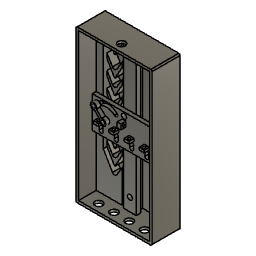
Progetto locker senza bottone v9 (Autodesk Fusion 360 design; units mm, degrees)
Autodesk Fusion 360 part; units mm, degrees
note: some values were not read from the file. Set by a fixed rule: which face or edge a step refers to.
sketch "Schizzo1" plane through (0, 0, 0) normal (0, 1, 0) x (1, 0, 0) in component "Scatola di fissaggio"
  line L0 (-30, -60) -> (30, -60)
  line L1 (30, -60) -> (30, 60)
  line L2 (30, 60) -> (-30, 60)
  line L3 (-30, 60) -> (-30, -60)
  point P0 (0, -60)
  point P1 (-30, 0)
  dimension "d1" = 60
  dimension "d2" = 120
  constraint horizontal L0
  constraint vertical L1
  constraint horizontal L2
  constraint vertical L3
  constraint midpoint L0 P0
  constraint midpoint L3 P1
  constraint vertical origin P0
  constraint horizontal origin P1
  measures "d1" distance of L0.start L0.end
  measures "d2" distance of L0.start L2.end
extrude "Estrusione1" add sketch "Schizzo1" along normal blind 22 makes body 1 in component "Scatola di fissaggio"
shell "Svuotamento1" thickness 2 removed faces 1 at (-10, 0, 20) on bodies 1 in component "Scatola di fissaggio"
ref_plane "Piano di lavoro1" through (0, 10, -58) normal (0, 0, 1) x (1, 0, 0) in component "Guida lineare"
sketch "Schizzo1 (2)" plane through (0, 12.5, -58) normal (0, 0, 1) x (1, 0, 0) in component "Guida lineare"
  line L0 (0, -26.6959) -> (0, 22.9147) construction
  line L1 (0, 0) -> (-5, 0)
  line L2 (-5, 0) -> (-5, 3.5)
  line L3 (-3.5, 5) -> (-2.5, 5)
  line L4 (-2.5, 5) -> (-2.5, 7.5)
  line L5 (28, 7.5) -> (-28, 7.5)
  line L6 (-5, 3.5) -> (-3.5, 5)
  line L7 (0, 0) -> (5, 0)
  line L8 (5, 0) -> (5, 3.5)
  line L9 (5, 3.5) -> (3.5, 5)
  line L10 (3.5, 5) -> (2.5, 5)
  line L11 (2.5, 5) -> (2.5, 7.5)
  point P0 (-5, 5)
  dimension "d7" = 2.5
  dimension "d8" = 5
  dimension "d9" = 5
  dimension "d10" = 2.5
  dimension "d11" = 1.5
  dimension "d12" = 1.5
  constraint vertical L0
  constraint coincident L1.start L0
  constraint coincident L0 L1.start
  constraint perpendicular L0 L1
  constraint perpendicular L1 L2
  constraint perpendicular L2 L3
  constraint perpendicular L3 L4
  constraint coincident L4.end L5
  constraint coincident P0 L2
  constraint coincident P0 L3
  constraint symmetric L0 L1.start L7.start
  constraint symmetric L0 L1.end L7.end
  constraint symmetric L0 L3.end L10.end
  constraint symmetric L0 L4.end L11.end
  constraint symmetric L0 L2.end L8.end
  constraint symmetric L0 L3.start L9.end
  measures "d7" distance of L3.end L4.end
  measures "d8" distance of L1.end P0
  measures "d9" distance of L1.start L1.end
  measures "d10" distance of L0 L4
  measures "d11" distance of P0 L2.end
  measures "d12" distance of P0 L3.start
extrude "Estrusione1'" add sketch "Schizzo1 (2)" along normal up to surface (116 mm away) separate body makes body 2 in component "Guida lineare"
sketch "Schizzo5" plane through (0, 0, 0) normal (0, 0, 1) x (1, 0, 0) in component "Base mobile"
  line L0 (5, 16) -> (3.5, 17.5)
  line L1 (5, 12.5) -> (5, 16)
  line L2 (0, 12.5) -> (5, 12.5)
  line L3 (0, -14.1959) -> (0, 35.4147)
  line L4 (0, 12) -> (5.5, 12)
  line L5 (5.5, 12) -> (5.5, 16.2071)
  line L6 (5.5, 16.2071) -> (3.8536, 17.8536)
  line L7 (3.8536, 17.8536) -> (6.8536, 17.8536)
  line L8 (6.8536, 17.8536) -> (6.8536, 10.8536)
  line L9 (6.8536, 10.8536) -> (0, 10.8536)
  line L10 (-6.8536, 10.8536) -> (0, 10.8536)
  line L11 (0, 12) -> (-5.5, 12)
  line L12 (-6.8536, 17.8536) -> (-6.8536, 10.8536)
  line L13 (-5.5, 12) -> (-5.5, 16.2071)
  line L14 (-5.5, 16.2071) -> (-3.8536, 17.8536)
  line L15 (-3.8536, 17.8536) -> (-6.8536, 17.8536)
  dimension "d135" = 0.5
  dimension "d196" = 3
  dimension "d197" = 7
  constraint horizontal L7
  constraint perpendicular L7 L8
  constraint coincident L3 L9.end
  constraint perpendicular L3 L9
  constraint symmetric L3 L4.start L11.start
  constraint symmetric L3 L4.end L11.end
  constraint symmetric L3 L5.end L13.end
  constraint symmetric L3 L6.end L14.end
  constraint symmetric L3 L7.end L12.start
  constraint symmetric L3 L8.end L10.start
  constraint symmetric L3 L9.end L10.end
  measures "d196" distance of L6.end L7.end
  measures "d197" distance of L7.end L8.end
extrude "Estrusione2" add sketch "Schizzo5" along normal mid plane 8 separate body makes body 3 in component "Base mobile"
sketch "Schizzo6" plane through (0, 10.8536, 0) normal (0, -1, 0) x (1, 0, 0) in component "Base mobile"
  line L0 (0.5, 5) -> (-0.5, 5)
  line L1 (-0.5, -5) -> (0.5, -5)
  line L2 (25, -12.5) -> (-25, -12.5)
  line L3 (-25, -12.5) -> (-25, 12.5)
  line L4 (-25, 12.5) -> (25, 12.5)
  line L5 (25, 12.5) -> (25, -12.5)
  line L6 (0.8536, -4) -> (0.8536, 4)
  line L7 (0.8536, 4) -> (-0.8536, 4)
  line L8 (-0.8536, 4) -> (-0.8536, -4)
  line L9 (-0.8536, -4) -> (0.8536, -4)
  point P0 (0, -12.5)
  point P1 (25, 0)
  dimension "d31" = 50
  dimension "d32" = 25
  constraint horizontal L2
  constraint vertical L3
  constraint horizontal L4
  constraint vertical L5
  constraint midpoint L2 P0
  constraint midpoint L5 P1
  constraint horizontal origin P1
  constraint vertical origin P0
  measures "d31" distance of L2.start L2.end
  measures "d32" distance of L2.start L4.end
extrude "Estrusione3" add sketch "Schizzo6" along normal blind 3 separate body contours L2 L3 L4 L5 | L6 L7 L8 L9 makes body 4 in component "Base mobile"
sketch "Schizzo3" plane through (0, 0, 60) normal (0, 0, 1) x (-1, 0, 0) in component "Scatola di fissaggio"
  line L0 (30, 0) -> (-30, 0)
  line L1 (-30, 0) -> (-30, -22)
  line L2 (-30, -22) -> (30, -22)
  line L3 (30, -22) -> (30, 0)
  circle A0 centre (0, -6) radius 3
  dimension "d82" = 6
  dimension "d83" = 6
  constraint vertical origin A0.centre
  measures "d82" diameter of A0
  measures "d83" distance of L0 A0.centre
extrude "Estrusione3'" cut sketch "Schizzo3" against normal up to surface (2 mm away) contours A0 bodies 1 in component "Scatola di fissaggio"
sketch "Schizzo4" plane through (0, 0, -60) normal (0, 0, -1) x (1, 0, 0) in component "Scatola di fissaggio"
  line L0 (30, 0) -> (-30, 0)
  line L1 (-30, 0) -> (-30, -22)
  line L2 (-30, -22) -> (30, -22)
  line L3 (30, -22) -> (30, 0)
  circle A0 centre (-18, -6) radius 3
  line L4 (-68.094, -6) -> (66.0156, -6) construction
  line L5 (0, 54.335) -> (0, -66.5386) construction
  circle A1 centre (-6, -6) radius 3
  circle A2 centre (18, -6) radius 3
  circle A3 centre (6, -6) radius 3
  dimension "d86" = 6
  dimension "d91" = 12
  dimension "d92" = 6
  dimension "d93" = 6
  dimension "d94" = 12
  dimension "d97" = 12
  constraint perpendicular L3 L4
  constraint perpendicular L0 L5
  constraint coincident A0.centre L4
  constraint coincident L4 A1.centre
  constraint symmetric A0 L5 A2
  constraint symmetric L5 A1 A3
  measures "d86" diameter of A0
  measures "d91" distance of L1 A0.centre
  measures "d92" distance of L0 L4
  measures "d93" diameter of A1
  measures "d94" distance of A0.centre A1.centre
  measures "d97" distance of L3 A2.centre
extrude "Estrusione4" cut sketch "Schizzo4" against normal up to surface (2 mm away) contours A0 | A1 | A2 | A3 bodies 1 in component "Scatola di fissaggio"
fillet "Raccordo1" radius 1 4 edges at (-30, 11, -60) (-30, 11, 60) (30, 11, 60) (30, 11, -60) on bodies 1 in component "Scatola di fissaggio"
sketch "Schizzo8" plane through (0, 7.8536, 0) normal (0, -1, 0) x (1, 0, 0) in component "Base mobile"
  line L0 (25, 12.5) -> (-25, 12.5)
  line L1 (-25, 12.5) -> (-25, -12.5)
  line L2 (-25, -12.5) -> (25, -12.5)
  line L3 (25, -12.5) -> (25, 12.5)
  circle A0 centre (0, 9.5) radius 2
  dimension "d101" = 4
  dimension "d102" = 3
  constraint vertical origin A0.centre
  measures "d101" diameter of A0
  measures "d102" distance of L0 A0.centre
extrude "Estrusione5" cut sketch "Schizzo8" against normal blind 3 contours A0 bodies 4 in component "Base mobile"
sketch "Schizzo5 (2)" plane through (0, 20, 0) normal (0, -1, 0) x (1, 0, 0) in component "Scatola di fissaggio"
  line L0 (-28, 58) -> (-28, -58)
  line L1 (-28, -58) -> (28, -58)
  line L2 (28, -58) -> (28, 58)
  line L3 (28, 58) -> (-28, 58)
  line L4 (-28, 58) -> (-7.5, 58)
  line L5 (-7.5, 58) -> (-7.5, -58)
  line L6 (-7.5, -58) -> (-28, -58)
  line L7 (-28, -58) -> (-28, 58)
  line L8 (-2.5, -58) -> (-2.5, 58)
  dimension "d106" = 5
  constraint horizontal L4
  constraint vertical L5
  constraint horizontal L6
  constraint vertical L7
  constraint coincident L1 L5.end
  constraint coincident L3 L0.start
  constraint collinear L0 L7
  measures "d106" distance of L5 L8
extrude "Estrusione5'" add sketch "Schizzo5 (2)" along normal blind 6 contours L0 L1 L3 L4 L5 L6 L7 bodies 1 in component "Scatola di fissaggio"
sketch "Schizzo6 (2)" plane through (0, 14, 0) normal (0, -1, 0) x (1, 0, 0) in component "Scatola di fissaggio"
  line L0 (-28, -58) -> (-7.5, -58)
  line L1 (-7.5, -58) -> (-7.5, 58)
  line L2 (-7.5, 58) -> (-28, 58)
  line L3 (-13.5, 41.6077) -> (-7.5, 52)
  line L4 (-13.5, 41.6077) -> (-19.5, 52)
  line L5 (-13.5, 29.6077) -> (-19.5, 40)
  line L6 (-13.5, 29.6077) -> (-7.5, 40)
  line L7 (-13.5, 17.6077) -> (-19.5, 28)
  line L8 (-13.5, 17.6077) -> (-7.5, 28)
  line L9 (-13.5, 5.6077) -> (-19.5, 16)
  line L10 (-13.5, 5.6077) -> (-7.5, 16)
  line L11 (-13.5, -6.3923) -> (-19.5, 4)
  line L12 (-13.5, -6.3923) -> (-7.5, 4)
  line L13 (-13.5, -18.3923) -> (-19.5, -8)
  line L14 (-13.5, -18.3923) -> (-7.5, -8)
  line L15 (-13.5, -30.3923) -> (-19.5, -20)
  line L16 (-13.5, -30.3923) -> (-7.5, -20)
  line L17 (-7.5, 40) -> (-7.5, 36)
  line L18 (-13.5, 25.6077) -> (-7.5, 36)
  line L19 (-13.5, 25.6077) -> (-19.5, 36)
  line L20 (-19.5, 40) -> (-19.5, 36)
  line L21 (-13.5, 13.6077) -> (-19.5, 24)
  line L22 (-13.5, 13.6077) -> (-7.5, 24)
  line L23 (-7.5, 28) -> (-7.5, 24)
  line L24 (-19.5, 28) -> (-19.5, 24)
  line L25 (-13.5, 1.6077) -> (-19.5, 12)
  line L26 (-13.5, 1.6077) -> (-7.5, 12)
  line L27 (-7.5, 16) -> (-7.5, 12)
  line L28 (-19.5, 16) -> (-19.5, 12)
  line L29 (-13.5, -10.3923) -> (-19.5, 0)
  line L30 (-13.5, -10.3923) -> (-7.5, 0)
  line L31 (-7.5, 4) -> (-7.5, 0)
  line L32 (-19.5, 4) -> (-19.5, 0)
  line L33 (-13.5, -22.3923) -> (-19.5, -12)
  line L34 (-13.5, -22.3923) -> (-7.5, -12)
  line L35 (-7.5, -8) -> (-7.5, -12)
  line L36 (-19.5, -8) -> (-19.5, -12)
  line L37 (-13.5, -34.3923) -> (-19.5, -24)
  line L38 (-13.5, -34.3923) -> (-7.5, -24)
  line L39 (-7.5, -20) -> (-7.5, -24)
  line L40 (-19.5, -20) -> (-19.5, -24)
  line L41 (-13.5, -46.3923) -> (-19.5, -36)
  line L42 (-13.5, -46.3923) -> (-7.5, -36)
  line L43 (-7.5, -32) -> (-7.5, -36)
  line L44 (-19.5, -32) -> (-19.5, -36)
  line L45 (-13.5, -42.3923) -> (-19.5, -32)
  line L46 (-13.5, -42.3923) -> (-7.5, -32)
  line L47 (-28, 58) -> (-28, -58)
  line L48 (-19.5, 58) -> (-19.5, -36)
  line L49 (-13.5, 58) -> (-13.5, -58) construction
  line L50 (-22.5, 58) -> (-22.5, -26.8038)
  line L51 (-22.5, -26.8038) -> (-19.5, -32)
  dimension "d110" = 60
  dimension "d113" = 0
  dimension "d114" = -12
  dimension "d115" = 4
  dimension "d116" = 60
  dimension "d119" = 12
  dimension "d120" = 0
  dimension "d124" = 12
  dimension "d125" = 6
  dimension "d126" = 6
  dimension "d128" = 3
  constraint coincident L1 L3.end
  constraint horizontal L3.end L4.end
  constraint coincident L1 L17.end
  constraint parallel L1 L17
  constraint horizontal L17.end L19.end
  constraint coincident L2 L48.start
  constraint vertical L48
  constraint coincident L4.end L48
  constraint coincident L2 L49.start
  constraint coincident L0 L49.end
  constraint perpendicular L0 L49
  constraint coincident L3.start L49
  constraint coincident L18.start L49
  constraint coincident L2 L50.start
  constraint perpendicular L2 L50
  constraint parallel L45 L51
  measures "d110" angle of L3 L4
  measures "d115" distance of L6.end L17.end
  measures "d116" angle of L18 L19
  measures "d124" distance of L1 L48
  measures "d125" distance of L1 L49
  measures "d126" distance of L1.end L3.end
  measures "d128" distance of L48 L50
extrude "Estrusione6" cut sketch "Schizzo6 (2)" against normal up to surface (6 mm away) contours L2 L20 L24 L28 L32 L36 L40 L48 L50 L51 | L1 L37 L38 L45 L46 L48 | L1 L3 L4 L5 L6 L48 | L1 L15 L16 L33 L34 L48 | L1 L7 L8 L18 L19 L48 | L1 L13 L14 L29 L30 L48 | L1 L9 L10 L21 L22 L48 | L1 L11 L12 L25 L26 L48 bodies 1 in component "Scatola di fissaggio"
fillet "Raccordo2" radius 2 7 edges at (-13.5, 17, 29.6077) (-13.5, 17, 17.6077) (-13.5, 17, 5.6077) (-13.5, 17, -6.3923) (-13.5, 17, -18.3923) (-13.5, 17, -30.3923) (-13.5, 17, -42.3923) on bodies 1 in component "Scatola di fissaggio"
sketch "Schizzo7" plane through (-25.0173, 0, -14.4437) normal (-0.866025, 0, -0.5) x (0, -1, 0) in component "Scatola di fissaggio"
  line L0 (-20, -11.0346) -> (-20, -23.0346)
  line L1 (-20, -23.0346) -> (-14, -23.0346)
  line L2 (-14, -23.0346) -> (-14, -11.0346)
  line L3 (-14, -11.0346) -> (-20, -11.0346)
  line L4 (-20, -11.0346) -> (-18, -23.0346)
  line L5 (-20, -23.0346) -> (-18, -23.0346)
  line L6 (-20, -23.0346) -> (-20, -11.0346)
  dimension "d131" = 2
  constraint coincident L0.start L3.end
  constraint coincident L1 L4.end
  constraint coincident L0.end L1.start
  measures "d131" distance of L0.end L4.end
extrude "Estrusione7" add sketch "Schizzo7" along normal up to surface (4 mm away) contours L0 L1 L4 L5 L6 bodies 1 in component "Scatola di fissaggio"
sketch "Schizzo2" plane through (0, 7.8536, 0) normal (0, -1, 0) x (1, 0, 0)
  circle A0 centre (0, 9.5) radius 2
  line L0 (25, 12.5) -> (-25, 12.5)
  line L1 (-25, 12.5) -> (-25, -12.5)
  line L2 (-25, -12.5) -> (25, -12.5)
  line L3 (25, -12.5) -> (25, 12.5)
sketch "Schizzo3 (2)" plane through (0, 7.8536, 0) normal (0, -1, 0) x (1, 0, 0)
sketch "Schizzo9" plane through (0, 7.8536, 0) normal (0, -1, 0) x (1, 0, 0) in component "Base mobile"
  line L0 (-22.5, -26.8038) -> (-22.5, 58)
  line L1 (-5, -58) -> (-5, 58)
  circle A0 centre (0, 9.5) radius 2
  line L2 (25, 12.5) -> (-25, 12.5)
  line L3 (-25, 12.5) -> (-25, -12.5)
  line L4 (-25, -12.5) -> (25, -12.5)
  line L5 (25, -12.5) -> (25, 12.5)
  line L6 (-0.8536, -4) -> (-0.8536, 4)
  circle A1 centre (0, 9.5) radius 2
  line L7 (-25, 12.5) -> (25, 12.5)
  line L8 (25, 12.5) -> (25, -12.5)
  line L9 (25, -12.5) -> (-25, -12.5)
  line L10 (-25, -12.5) -> (-25, 12.5)
  arc A2 (-22.0425, 8.5785) -> (-19.9575, 6.4215) centre (-21, 7.5) ccw
  arc A3 (-7.5425, 6.4215) -> (-5.4575, 8.5785) centre (-6.5, 7.5) ccw
  arc A4 (-7.5425, 6.4215) -> (-19.9575, 6.4215) centre (-13.75, 0) ccw
  arc A5 (-5.4575, 8.5785) -> (-22.0425, 8.5785) centre (-13.75, 0) ccw
  circle A6 centre (-13.75, 0) radius 1.5
  dimension "d138" = 5
  dimension "d139" = 3
  dimension "d140" = 3
  constraint equal A2 A3
  constraint tangent L0 A2
  constraint tangent L1 A3
  constraint horizontal A3.centre A2.centre
  constraint tangent A2 A4
  constraint concentric A4 A5
  constraint tangent A3 A4
  constraint tangent A2 A5
  constraint horizontal origin A4.centre
  constraint concentric A5 A6
  measures "d138" distance of A2.centre L7
  measures "d139" diameter of A2
  measures "d140" diameter of A6
extrude "Estrusione6'" cut sketch "Schizzo9" against normal up to surface (3 mm away) contours A2 A3 A4 A5 | A6 bodies 4 in component "Base mobile"
sketch "Schizzo1 (3)" plane through (0, 7.8536, 0) normal (0, -1, 0) x (1, 0, 0) in component "Perno rotante"
  circle A0 centre (-13.75, 0) radius 1.5
  circle A1 centre (-21, 7.5) radius 1.5
  arc A2 (-22.0425, 8.5785) -> (-19.9575, 6.4215) centre (-21, 7.5) ccw
  line L0 (-14.6235, 2.3424) -> (-18.6885, 6.5476)
  line L1 (-21, 7.5) -> (-13.75, 0) construction
  line L2 (-16.0615, 0.9524) -> (-20.1265, 5.1576)
  arc A3 (-18.6885, 6.5476) -> (-20.1265, 5.1576) centre (-21, 7.5) ccw
  arc A4 (-16.0615, 0.9524) -> (-14.6235, 2.3424) centre (-13.75, 0) ccw
  dimension "d143" = 5
  dimension "d144" = 3
  dimension "d145" = 5
  dimension "d147" = 1
  constraint concentric A1 A3
  constraint coincident A0.centre L1.end
  constraint coincident A1.centre A2.centre
  constraint parallel L1 L2
  constraint parallel L0 L1
  constraint symmetric L0 L1 L2
  measures "d143" diameter of A4
  measures "d144" diameter of A1
  measures "d145" diameter of A3
  measures "d147" distance of L1 L2
extrude "Estrusione1''" add sketch "Schizzo1 (3)" along normal blind 3 separate body makes body 5 in component "Perno rotante"
sketch "Schizzo4 (2)" plane through (0, 0, 0) normal (0, 0, 1) x (1, 0, 0)
  circle A0 centre (-18, 6) radius 3 construction
  circle A1 centre (-6, 6) radius 3 construction
  circle A2 centre (6, 6) radius 3 construction
  circle A3 centre (18, 6) radius 3 construction
sketch "Schizzo10" plane through (0, 7.8536, 0) normal (0, -1, 0) x (1, 0, 0) in component "Base mobile"
  line L0 (-18, 0) -> (-18, -10.4085) construction
  line L1 (-6, 0) -> (-6, -9.9815) construction
  line L2 (6, 0) -> (6, -9.9815) construction
  line L3 (18, 0) -> (18, -9.9815) construction
  line L4 (-25, -12.5) -> (25, -12.5)
  line L5 (-19.5, -9.5) -> (-19.5, -6.5)
  line L6 (-16.5, -9.5) -> (-16.5, -6.5)
  arc A0 (-16.5, -6.5) -> (-19.5, -6.5) centre (-18, -6.5) ccw
  arc A1 (-19.5, -9.5) -> (-16.5, -9.5) centre (-18, -9.5) ccw
  line L7 (-12, 0.0355) -> (-12, -13.6259) construction
  arc A2 (-4.5, -6.5) -> (-7.5, -6.5) centre (-6, -6.5) ccw
  line L8 (-4.5, -9.5) -> (-4.5, -6.5)
  line L9 (-7.5, -9.5) -> (-7.5, -6.5)
  arc A3 (-7.5, -9.5) -> (-4.5, -9.5) centre (-6, -9.5) ccw
  line L10 (0, 0) -> (0, -13.6833) construction
  line L11 (16.5, -9.5) -> (16.5, -6.5)
  arc A4 (19.5, -6.5) -> (16.5, -6.5) centre (18, -6.5) ccw
  line L12 (19.5, -9.5) -> (19.5, -6.5)
  arc A5 (16.5, -9.5) -> (19.5, -9.5) centre (18, -9.5) ccw
  line L13 (4.5, -9.5) -> (4.5, -6.5)
  arc A6 (7.5, -6.5) -> (4.5, -6.5) centre (6, -6.5) ccw
  line L14 (7.5, -9.5) -> (7.5, -6.5)
  arc A7 (4.5, -9.5) -> (7.5, -9.5) centre (6, -9.5) ccw
  point P0 (-18, 0)
  point P1 (-6, 0)
  point P2 (6, 0)
  point P3 (18, 0)
  dimension "d150" = 3
  dimension "d151" = 3
  dimension "d154" = 3
  constraint coincident P0 L0.start
  constraint vertical L0
  constraint coincident P1 L1.start
  constraint vertical L1
  constraint coincident P2 L2.start
  constraint vertical L2
  constraint coincident P3 L3.start
  constraint vertical L3
  constraint coincident L0 A1.centre
  constraint tangent L5 A1
  constraint parallel L0 L6
  constraint coincident L0 A0.centre
  constraint tangent L6 A0
  constraint tangent L5 A0
  constraint equal A0 A1
  constraint perpendicular L4 L7
  constraint symmetric L5.start L7 L8.start
  constraint symmetric L5.end L7 A2.start
  constraint symmetric L6.start L7 L9.start
  constraint symmetric L6.end L7 A2.end
  constraint symmetric A0 L7 A2
  constraint symmetric A1 L7 A3
  constraint coincident L10.start origin
  constraint perpendicular L4 L10
  constraint symmetric L5.start L10 L12.start
  constraint symmetric L5.end L10 A4.start
  constraint symmetric L6.start L10 L11.start
  constraint symmetric L6.end L10 L11.end
  constraint symmetric A0 L10 A4
  constraint symmetric A1 L10 A5
  constraint symmetric A2.end L10 A6.start
  constraint symmetric A2.start L10 L13.end
  constraint symmetric A2 L10 A6
  constraint symmetric L8.start L10 L13.start
  constraint symmetric L9.start L10 L14.start
  constraint symmetric A3 L10 A7
  measures "d150" diameter of A1
  measures "d151" distance of A1.centre L4
  measures "d154" distance of A1.centre A0.centre
extrude "Estrusione7'" cut sketch "Schizzo10" against normal up to surface (3 mm away) bodies 4 in component "Base mobile"
sketch "Schizzo5 (3)" plane through (0, 7.8536, 0) normal (0, -1, 0) x (1, 0, 0)
  line L0 (-7.5, -9.5) -> (-7.5, -6.5)
  arc A0 (-4.5, -6.5) -> (-7.5, -6.5) centre (-6, -6.5) ccw
  line L1 (-4.5, -6.5) -> (-4.5, -9.5)
  arc A1 (-7.5, -9.5) -> (-4.5, -9.5) centre (-6, -9.5) ccw
  line L2 (4.5, -9.5) -> (4.5, -6.5)
  arc A2 (7.5, -6.5) -> (4.5, -6.5) centre (6, -6.5) ccw
  line L3 (7.5, -6.5) -> (7.5, -9.5)
  arc A3 (4.5, -9.5) -> (7.5, -9.5) centre (6, -9.5) ccw
  line L4 (-19.5, -9.5) -> (-19.5, -6.5)
  arc A4 (-16.5, -6.5) -> (-19.5, -6.5) centre (-18, -6.5) ccw
  line L5 (-16.5, -6.5) -> (-16.5, -9.5)
  arc A5 (-19.5, -9.5) -> (-16.5, -9.5) centre (-18, -9.5) ccw
  line L6 (16.5, -9.5) -> (16.5, -6.5)
  arc A6 (19.5, -6.5) -> (16.5, -6.5) centre (18, -6.5) ccw
  line L7 (19.5, -6.5) -> (19.5, -9.5)
  arc A7 (16.5, -9.5) -> (19.5, -9.5) centre (18, -9.5) ccw
  arc A8 (-7.5425, 6.4215) -> (-19.9575, 6.4215) centre (-13.75, 0) ccw
  arc A9 (-22.0425, 8.5785) -> (-19.9575, 6.4215) centre (-21, 7.5) ccw
  arc A10 (-5.4575, 8.5785) -> (-22.0425, 8.5785) centre (-13.75, 0) ccw
  arc A11 (-7.5425, 6.4215) -> (-5.4575, 8.5785) centre (-6.5, 7.5) ccw
  circle A12 centre (-13.75, 0) radius 1.5
  circle A13 centre (0, 9.5) radius 2
  line L8 (25, 12.5) -> (-25, 12.5)
  line L9 (-25, 12.5) -> (-25, -12.5)
  line L10 (-25, -12.5) -> (25, -12.5)
  line L11 (25, -12.5) -> (25, 12.5)
  line L12 (-1.5, 7) -> (1.5, 7)
  line L13 (1.5, 7) -> (1.5, 3)
  line L14 (1.5, 3) -> (-1.5, 3)
  line L15 (-1.5, 3) -> (-1.5, 7)
  line L16 (0, 12.5) -> (0, -12.5) construction
  line L17 (-20, -1.5) -> (-16, -1.5)
  line L18 (-16, -1.5) -> (-16, -3.5)
  line L19 (-16, -3.5) -> (-20, -3.5)
  line L20 (-20, -3.5) -> (-20, -1.5)
  line L21 (25, -12.5) -> (-25, -12.5)
  line L22 (-18, 0) -> (-18, -10.4085)
  line L23 (-6, 0) -> (-6, -9.9815)
  line L24 (6, 0) -> (6, -9.9815)
  line L25 (18, 0) -> (18, -9.9815)
  line L26 (-12, 0.0355) -> (-12, -13.6259)
  line L27 (0, 0) -> (0, -13.6833)
  line L28 (-4, -1.5) -> (-8, -1.5)
  line L29 (-4, -3.5) -> (-4, -1.5)
  line L30 (-8, -3.5) -> (-4, -3.5)
  line L31 (-8, -1.5) -> (-8, -3.5)
  line L32 (8, -1.5) -> (8, -3.5)
  line L33 (8, -3.5) -> (4, -3.5)
  line L34 (4, -3.5) -> (4, -1.5)
  line L35 (4, -1.5) -> (8, -1.5)
  line L36 (20, -3.5) -> (20, -1.5)
  line L37 (16, -3.5) -> (20, -3.5)
  line L38 (16, -1.5) -> (16, -3.5)
  line L39 (20, -1.5) -> (16, -1.5)
  dimension "d155" = 4
  dimension "d156" = 3
  dimension "d157" = 5.5
  dimension "d158" = 4
  dimension "d159" = 5
  dimension "d160" = 2
  dimension "d161" = 9
  constraint horizontal L12
  constraint vertical L13
  constraint horizontal L14
  constraint vertical L15
  constraint midpoint L8 L16.start
  constraint midpoint L10 L16.end
  constraint symmetric L13 L15 L16
  constraint horizontal L17
  constraint vertical L18
  constraint horizontal L19
  constraint vertical L20
  constraint symmetric L17.start L26 L28.start
  constraint symmetric L17.end L26 L28.end
  constraint symmetric L18.end L26 L30.start
  constraint symmetric L19.end L26 L29.start
  constraint symmetric L16 L17.start L36.end
  constraint symmetric L16 L17.end L38.start
  constraint symmetric L16 L18.end L37.start
  constraint symmetric L16 L19.end L36.start
  constraint symmetric L16 L28.start L34.end
  constraint symmetric L16 L28.end L32.start
  constraint symmetric L16 L29.start L33.end
  constraint symmetric L16 L30.start L32.end
  measures "d155" distance of L12.start L14.end
  measures "d156" distance of L13.end L14.end
  measures "d157" distance of L12 L16.start
  measures "d158" distance of L17.start L17.end
  measures "d159" distance of L9 L20
  measures "d160" distance of L17.start L19.end
  measures "d161" distance of L19 L21
extrude "Estrusione8" add sketch "Schizzo5 (3)" along normal blind 4 contours L12 L13 L14 L15 | L17 L19 L20 L22 | L17 L18 L19 L22 | L23 L28 L29 L30 | L23 L28 L30 L31 | L24 L32 L33 L35 | L24 L33 L34 L35 | L25 L36 L37 L39 | L25 L37 L38 L39 bodies 4 in component "Base mobile"
sketch "Schizzo6 (3)" plane through (0, 0, -3.5) normal (0, 0, -1) x (1, 0, 0)
  line L0 (-20, -7.8536) -> (-16, -7.8536)
  line L1 (-16, -7.8536) -> (-16, -3.8536)
  line L2 (-16, -3.8536) -> (-20, -3.8536)
  line L3 (-20, -3.8536) -> (-20, -7.8536)
  circle A0 centre (-18, -5.8536) radius 1
  circle A1 centre (-6, -5.8536) radius 1
  circle A2 centre (6, -5.8536) radius 1
  circle A3 centre (18, -5.8536) radius 1
  line L4 (-8, -7.8536) -> (-8, -3.8536)
  line L5 (4, -7.8536) -> (4, -3.8536)
  line L6 (16, -7.8536) -> (16, -3.8536)
  dimension "d164" = 2
  dimension "d165" = 2
  dimension "d166" = 2
  dimension "d167" = 2
  dimension "d168" = 2
  dimension "d169" = 2
  constraint equal A0 A1
  constraint equal A1 A2
  constraint equal A2 A3
  constraint horizontal A0.centre A1.centre
  constraint horizontal A1.centre A2.centre
  constraint horizontal A2.centre A3.centre
  measures "d164" diameter of A0
  measures "d165" distance of L3 A0.centre
  measures "d166" distance of L2 A0.centre
  measures "d167" distance of A1.centre L4
  measures "d168" distance of A2.centre L5
  measures "d169" distance of A3.centre L6
extrude "Estrusione9" cut sketch "Schizzo6 (3)" against normal up to surface (2 mm away) contours A0 | A1 | A2 | A3 bodies 4 in component "Base mobile"
sketch "Schizzo7 (2)" plane through (-1.5, 0, 0) normal (-1, 0, 0) x (0, -1, 0)
  line L0 (-7.8536, 7) -> (-7.8536, 3)
  line L1 (-7.8536, 3) -> (-3.8536, 3)
  line L2 (-3.8536, 3) -> (-3.8536, 7)
  line L3 (-3.8536, 7) -> (-7.8536, 7)
  circle A0 centre (-5.8536, 5) radius 1
  dimension "d172" = 2
  dimension "d173" = 2
  dimension "d174" = 2
  measures "d172" diameter of A0
  measures "d173" distance of L2 A0.centre
  measures "d174" distance of L1 A0.centre
extrude "Estrusione10" cut sketch "Schizzo7 (2)" against normal blind 3 contours A0 bodies 4 in component "Base mobile"
sketch "Schizzo8 (2)" plane through (0, 10.8536, 0) normal (0, 1, 0) x (-1, 0, 0)
  line L0 (7.5, -6.5) -> (7.5, -9.5)
  arc A0 (4.5, -9.5) -> (7.5, -9.5) centre (6, -9.5) ccw
  line L1 (4.5, -9.5) -> (4.5, -6.5)
  arc A1 (7.5, -6.5) -> (4.5, -6.5) centre (6, -6.5) ccw
  line L2 (-4.5, -6.5) -> (-4.5, -9.5)
  arc A2 (-7.5, -9.5) -> (-4.5, -9.5) centre (-6, -9.5) ccw
  line L3 (-7.5, -9.5) -> (-7.5, -6.5)
  arc A3 (-4.5, -6.5) -> (-7.5, -6.5) centre (-6, -6.5) ccw
  line L4 (19.5, -6.5) -> (19.5, -9.5)
  arc A4 (16.5, -9.5) -> (19.5, -9.5) centre (18, -9.5) ccw
  line L5 (16.5, -9.5) -> (16.5, -6.5)
  arc A5 (19.5, -6.5) -> (16.5, -6.5) centre (18, -6.5) ccw
  line L6 (-16.5, -6.5) -> (-16.5, -9.5)
  arc A6 (-19.5, -9.5) -> (-16.5, -9.5) centre (-18, -9.5) ccw
  line L7 (-19.5, -9.5) -> (-19.5, -6.5)
  arc A7 (-16.5, -6.5) -> (-19.5, -6.5) centre (-18, -6.5) ccw
  arc A8 (19.9575, 6.4215) -> (7.5425, 6.4215) centre (13.75, 0) ccw
  arc A9 (5.4575, 8.5785) -> (7.5425, 6.4215) centre (6.5, 7.5) ccw
  arc A10 (22.0425, 8.5785) -> (5.4575, 8.5785) centre (13.75, 0) ccw
  arc A11 (19.9575, 6.4215) -> (22.0425, 8.5785) centre (21, 7.5) ccw
  circle A12 centre (13.75, 0) radius 1.5
  circle A13 centre (0, 9.5) radius 2
  line L8 (25, 12.5) -> (-25, 12.5)
  line L9 (-25, 12.5) -> (-25, -12.5)
  line L10 (-25, -12.5) -> (25, -12.5)
  line L11 (25, -12.5) -> (25, 12.5)
  line L12 (-12, 4.5) -> (-20, 4.5)
  line L13 (-20, 4.5) -> (-20, 8.5)
  line L14 (-20, 8.5) -> (-12, 8.5)
  line L15 (-12, 8.5) -> (-12, 4.5)
  dimension "d177" = 8
  dimension "d178" = 4
  dimension "d179" = 5
  dimension "d180" = 4
  constraint horizontal L12
  constraint vertical L13
  constraint horizontal L14
  constraint vertical L15
  measures "d177" distance of L12.start L12.end
  measures "d178" distance of L12.start L14.end
  measures "d179" distance of L9 L13
  measures "d180" distance of L8 L14
extrude "Estrusione11" add sketch "Schizzo8 (2)" along normal blind 5 contours L12 L13 L14 L15 bodies 4 in component "Base mobile"
sketch "Schizzo9 (2)" plane through (0, 0, 4.5) normal (0, 0, -1) x (1, 0, 0)
  line L0 (20, -10.8536) -> (12, -10.8536)
  line L1 (12, -10.8536) -> (12, -15.8536)
  line L2 (12, -15.8536) -> (20, -15.8536)
  line L3 (20, -15.8536) -> (20, -10.8536)
  circle A0 centre (16, -13.8536) radius 1
  dimension "d183" = 2
  dimension "d184" = 4
  dimension "d185" = 2
  measures "d183" diameter of A0
  measures "d184" distance of L3 A0.centre
  measures "d185" distance of L2 A0.centre
extrude "Estrusione12" cut sketch "Schizzo9 (2)" against normal up to surface (4 mm away) contours A0 bodies 4 in component "Base mobile"
sketch "Schizzo2 (2)" plane through (0, 12.5, 0) normal (0, -1, 0) x (1, 0, 0) in component "Guida lineare"
  line L0 (5, 58) -> (-5, 58)
  line L1 (-5, 58) -> (-5, -58)
  line L2 (-5, -58) -> (5, -58)
  line L3 (5, -58) -> (5, 58)
  circle A0 centre (0, 48) radius 2
  circle A1 centre (0, -48) radius 2
  dimension "d188" = 4
  dimension "d189" = 4
  dimension "d190" = 10
  dimension "d191" = 10
  constraint vertical origin A1.centre
  constraint vertical origin A0.centre
  measures "d188" diameter of A0
  measures "d189" diameter of A1
  measures "d190" distance of L2 A1.centre
  measures "d191" distance of L0 A0.centre
extrude "Estrusione2'" cut sketch "Schizzo2 (2)" against normal up to surface (7.5 mm away) contours A0 | A1 bodies 2 in component "Guida lineare"
sketch "Schizzo8 (3)" plane through (0, 20, 0) normal (0, -1, 0) x (1, 0, 0) in component "Scatola di fissaggio"
  arc A0 (-15.2321, 32.6077) -> (-11.7679, 32.6077) centre (-13.5, 33.6077) ccw
  line L0 (-11.7679, 32.6077) -> (-7.5, 40)
  line L1 (-7.5, 40) -> (-7.5, 36)
  line L2 (-7.5, 36) -> (-13.5, 25.6077)
  line L3 (-13.5, 25.6077) -> (-19.5, 36)
  line L4 (-19.5, 36) -> (-19.5, 40)
  line L5 (-19.5, 40) -> (-15.2321, 32.6077)
  arc A1 (-15.2321, 20.6077) -> (-11.7679, 20.6077) centre (-13.5, 21.6077) ccw
  line L6 (-11.7679, 20.6077) -> (-7.5, 28)
  line L7 (-7.5, 28) -> (-7.5, 24)
  line L8 (-7.5, 24) -> (-13.5, 13.6077)
  line L9 (-13.5, 13.6077) -> (-19.5, 24)
  line L10 (-19.5, 24) -> (-19.5, 28)
  line L11 (-19.5, 28) -> (-15.2321, 20.6077)
  arc A2 (-15.2321, 8.6077) -> (-11.7679, 8.6077) centre (-13.5, 9.6077) ccw
  line L12 (-11.7679, 8.6077) -> (-7.5, 16)
  line L13 (-7.5, 16) -> (-7.5, 12)
  line L14 (-7.5, 12) -> (-13.5, 1.6077)
  line L15 (-13.5, 1.6077) -> (-19.5, 12)
  line L16 (-19.5, 12) -> (-19.5, 16)
  line L17 (-19.5, 16) -> (-15.2321, 8.6077)
  arc A3 (-15.2321, -3.3923) -> (-11.7679, -3.3923) centre (-13.5, -2.3923) ccw
  line L18 (-11.7679, -3.3923) -> (-7.5, 4)
  line L19 (-7.5, 4) -> (-7.5, 0)
  line L20 (-7.5, 0) -> (-13.5, -10.3923)
  line L21 (-13.5, -10.3923) -> (-19.5, 0)
  line L22 (-19.5, 0) -> (-19.5, 4)
  line L23 (-19.5, 4) -> (-15.2321, -3.3923)
  arc A4 (-15.2321, -15.3923) -> (-11.7679, -15.3923) centre (-13.5, -14.3923) ccw
  line L24 (-11.7679, -15.3923) -> (-7.5, -8)
  line L25 (-7.5, -8) -> (-7.5, -12)
  line L26 (-7.5, -12) -> (-13.5, -22.3923)
  line L27 (-13.5, -22.3923) -> (-19.5, -12)
  line L28 (-19.5, -12) -> (-19.5, -8)
  line L29 (-19.5, -8) -> (-15.2321, -15.3923)
  line L30 (-13.5, -34.3923) -> (-16.9641, -36.3923)
  line L31 (-16.9641, -36.3923) -> (-15.2321, -39.3923)
  arc A5 (-15.2321, -39.3923) -> (-11.7679, -39.3923) centre (-13.5, -38.3923) ccw
  line L32 (-11.7679, -39.3923) -> (-7.5, -32)
  line L33 (-7.5, -32) -> (-7.5, -58)
  line L34 (-7.5, -58) -> (28, -58)
  line L35 (28, -58) -> (28, 58)
  line L36 (28, 58) -> (-7.5, 58)
  line L37 (-7.5, 58) -> (-7.5, 52)
  line L38 (-7.5, 52) -> (-13.5, 41.6077)
  line L39 (-13.5, 41.6077) -> (-19.5, 52)
  line L40 (-19.5, 52) -> (-19.5, 58)
  line L41 (-19.5, 58) -> (-22.5, 58)
  line L42 (-22.5, 58) -> (-22.5, -25.7321)
  line L43 (-22.5, -25.7321) -> (-19.5, -24)
  line L44 (-19.5, -24) -> (-19.5, -20)
  line L45 (-19.5, -20) -> (-15.2321, -27.3923)
  arc A6 (-15.2321, -27.3923) -> (-11.7679, -27.3923) centre (-13.5, -26.3923) ccw
  line L46 (-11.7679, -27.3923) -> (-7.5, -20)
  line L47 (-7.5, -20) -> (-7.5, -24)
  line L48 (-7.5, -24) -> (-13.5, -34.3923)
  circle A7 centre (0, 48) radius 2
  circle A8 centre (0, -48) radius 2
extrude "Estrusione8'" cut sketch "Schizzo8 (3)" against normal up to surface (2 mm away) contours A7 | A8 bodies 1 in component "Scatola di fissaggio"
component "Scatola di fissaggio" placed x (1, 0, 0) y (0, 1, 0) z (0, 0, 1) at (0, 0, 0)
component "Guida lineare" placed x (1, 0, 0) y (0, 1, 0) z (0, 0, 1) at (0, 0, 0)
component "Base mobile" placed x (1, 0, 0) y (0, 1, 0) z (0, 0, 1) at (0, 0, 0)
component "Perno rotante" placed x (1, 0, 0) y (0, 1, 0) z (0, 0, 1) at (0, 0, 0)
equation "d12 = d11"
